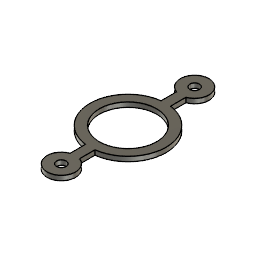
Ring2 (Autodesk Fusion 360 design; units mm, degrees)
part number: 2026-03-12-21-02-53-361
Autodesk Fusion 360 part; units mm, degrees
note: some values were not read from the file. Set by a fixed rule: which sketch regions a step uses.
sketch "Sketch1" plane through (0, 0, 0) normal (0, 0, 1) x (1, 0, 0)
  circle A0 centre (0, 0) radius 90
  circle A1 centre (0, 65) radius 10
  circle A2 centre (0, -65) radius 10
  circle A3 centre (0, 0) radius 25
  circle A4 centre (0, 0) radius 35
  circle A5 centre (0, 65) radius 20
  circle A6 centre (0, -65) radius 20
  line L0 (-10, 30) -> (10, 30)
  line L1 (10, 30) -> (10, 50)
  line L2 (10, 50) -> (-10, 50)
  line L3 (-10, 50) -> (-10, 30)
  line L4 (-10, -30) -> (10, -30)
  line L5 (10, -30) -> (10, -50)
  line L6 (10, -50) -> (-10, -50)
  line L7 (-10, -50) -> (-10, -30)
  dimension "d1" = 50
  constraint coincident A0.centre A3.centre
  constraint concentric A1 A5
  constraint concentric A2 A6
  constraint horizontal L0
  constraint vertical L1
  constraint horizontal L2
  constraint vertical L3
  constraint horizontal L4
  constraint vertical L5
  constraint horizontal L6
  constraint vertical L7
  measures "d1" diameter of A3
sketch "Sketch2" plane through (0, 0, 0) normal (0, 0, 1) x (1, 0, 0)
sketch "Sketch3" plane through (0, 0, 0) normal (0, 0, 1) x (1, 0, 0)
  circle A0 centre (0, 0) radius 30
  constraint coincident A0.centre origin
sketch "Sketch4" plane through (0, 0, 0) normal (0, 0, 1) x (1, 0, 0)
sketch "Sketch5" plane through (0, 0, 0) normal (0, 1, 0) x (1, 0, 0)
sketch "Sketch6" plane through (0, 0, 0) normal (0, 0, 1) x (1, 0, 0)
  circle A0 centre (0, 65) radius 5.25
  circle A1 centre (0, 65) radius 10
  dimension "d6" = 10.5
  constraint concentric A0 A1
  measures "d6" diameter of A0
sketch "Sketch7" plane through (0, 0, 0) normal (0, 0, 1) x (1, 0, 0)
  circle A0 centre (0, -65) radius 5.25
  circle A1 centre (0, -65) radius 10
  dimension "d9" = 10.5
  constraint concentric A0 A1
  measures "d9" diameter of A0
sketch "Sketch8" plane through (0, 0, 0) normal (0, 0, 1) x (1, 0, 0)
  circle A0 centre (0, 0) radius 40
  circle A1 centre (0, 0) radius 30
  circle A2 centre (0, 0) radius 30
  constraint coincident A0.centre A1.centre
  constraint concentric A0 A1
  constraint concentric A0 A2
sketch "Sketch9" plane through (0, 0, 0) normal (0, 0, 1) x (1, 0, 0)
sketch "Sketch10" plane through (0, 0, 0) normal (0, 0, 1) x (1, 0, 0)
sketch "Sketch11" plane through (0, 0, 0) normal (0, 0, 1) x (1, 0, 0)
sketch "Sketch12" plane through (0, 0, 0) normal (0, 0, 1) x (1, 0, 0)
  circle A0 centre (0, 65) radius 15
  circle A1 centre (0, 65) radius 20
  constraint concentric A0 A1
sketch "Sketch13" plane through (0, 0, 0) normal (0, 0, 1) x (1, 0, 0)
  circle A0 centre (0, -65) radius 15
  circle A1 centre (0, -65) radius 20
  constraint concentric A0 A1
extrude "Extrude7" cut sketch "Sketch13" along normal blind 22
sketch "Sketch14" plane through (0, 0, 0) normal (0, 0, 1) x (1, 0, 0)
  line L0 (-10, -35) -> (10, -35)
  line L1 (10, -35) -> (10, -59)
  line L2 (10, -59) -> (-10, -59)
  line L3 (-10, -59) -> (-10, -35)
  line L4 (-10, 35) -> (10, 35)
  line L5 (10, 35) -> (10, 58)
  line L6 (10, 58) -> (-10, 58)
  line L7 (-10, 58) -> (-10, 35)
  constraint horizontal L0
  constraint vertical L1
  constraint horizontal L2
  constraint vertical L3
  constraint horizontal L4
  constraint vertical L5
  constraint horizontal L6
  constraint vertical L7
sketch "Sketch15" plane through (0, 0, 0) normal (0, 0, 1) x (1, 0, 0)
sketch "Sketch16" plane through (0, 0, 0) normal (0, 0, 1) x (1, 0, 0)
sketch "Sketch17" plane through (0, 0, 0) normal (0, 0, 1) x (1, 0, 0)
sketch "Sketch18" plane through (0, 0, 0) normal (0, 0, 1) x (1, 0, 0)
  line L0 (0, -60) -> (0, 60)
  circle A0 centre (0, 0) radius 40
  circle A1 centre (0, 0) radius 30
  circle A2 centre (0, 70) radius 5
  circle A3 centre (0, -70) radius 5
  circle A4 centre (0, 70) radius 15
  circle A5 centre (0, -70) radius 15
  constraint vertical L0
  constraint coincident A0.centre A1.centre
  constraint concentric A0 A1
  constraint concentric A2 A4
  constraint concentric A3 A5
sketch "Sketch19" plane through (0, 0, 0) normal (0, 0, 1) x (1, 0, 0)
extrude "Extrude9" add sketch "Sketch18" along normal blind 5 separate body contours L0 A0 A1 | L0 A0 A1 | A4 | A5 makes body 1 at (11.5922, -69.0064, 5) makes body 2 at (36.4061, 3.4777, 5) makes body 3 at (11.6108, 69.2548, 0)
sketch "Sketch20" plane through (0, 0, 0) normal (0, 0, 1) x (1, 0, 0)
  line L0 (-7, -37) -> (8, -37)
  line L1 (8, -37) -> (8, -59)
  line L2 (8, -59) -> (-7, -59)
  line L3 (-7, -59) -> (-7, -37)
  line L4 (8, -37) -> (-8, -37)
  line L5 (-8, -37) -> (-8, -59)
  line L6 (-8, -59) -> (8, -59)
  line L7 (8, -59) -> (8, -37)
  line L8 (-8, 37) -> (7, 37)
  line L9 (7, 37) -> (7, 61)
  line L10 (7, 61) -> (-8, 61)
  line L11 (-8, 61) -> (-8, 37)
  line L12 (-5, 38) -> (5, 38)
  line L13 (5, 38) -> (5, 59)
  line L14 (5, 59) -> (-5, 59)
  line L15 (-5, 59) -> (-5, 38)
  line L16 (5, -35) -> (-5, -35)
  line L17 (-5, -35) -> (-5, -59)
  line L18 (-5, -59) -> (5, -59)
  line L19 (5, -59) -> (5, -35)
  constraint horizontal L0
  constraint vertical L1
  constraint horizontal L2
  constraint vertical L3
  constraint horizontal L4
  constraint vertical L5
  constraint horizontal L6
  constraint vertical L7
  constraint horizontal L8
  constraint vertical L9
  constraint horizontal L10
  constraint vertical L11
  constraint horizontal L12
  constraint vertical L13
  constraint horizontal L14
  constraint vertical L15
  constraint horizontal L16
  constraint vertical L17
  constraint horizontal L18
  constraint vertical L19
  constraint coincident L2 L17.end
extrude "Extrude10" add sketch "Sketch20" along normal blind 5 contours L0 L2 L4 L6 L17 L18 L19 | L12 L13 L14 L15 bodies 1 2 3
